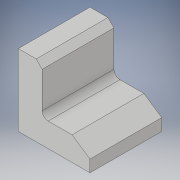
# Autodesk Inventor part: Chamfer
Saved by Autodesk Inventor 2017 (Build 210142000, 142)
## iProperties
Created: 2020-02-03
Part Number: Chamfer
Material: Generic
Document SubType Name: Modeling
Designer: 10042265
Density: 1 g/cm^3
Appearance: Default
Author: 10042265
Autodesk Inventor part; units mm, degrees
ref_plane "YZ Plane" through (0, 0, 0) normal (1, 0, 0) x (0, 1, 0)
ref_plane "XZ Plane" through (0, 0, 0) normal (0, 1, 0) x (-1, 0, 0)
ref_plane "XY Plane" through (0, 0, 0) normal (0, 0, 1) x (1, 0, 0)
sketch "Sketch1" plane through (0, 0, 0) normal (0, 0, 1) x (1, 0, 0)
  line L0 (0, 0) -> (38.1, 0)
  line L1 (38.1, 0) -> (38.1, 12.7)
  line L2 (38.1, 12.7) -> (12.7, 12.7)
  line L3 (12.7, 12.7) -> (12.7, 38.1)
  line L4 (12.7, 38.1) -> (0, 38.1)
  line L5 (0, 38.1) -> (0, 0)
  dimension "d0" = 38.1
  dimension "d1" = 12.7
  dimension "d2" = 25.4
  dimension "d3" = 25.4
  constraints: 12 end point, 4 perpendicular, 1 horizontal, 1 vertical
  measures "d0" distance of L0.start L0.end
  measures "d1" distance of L0.end L1.end
  measures "d2" distance of L1.end L2.end
  measures "d3" distance of L2.end L3.end
extrude "Extrusion1" add sketch "Sketch1" along normal blind 38.1
fillet "Fillet3" radius 3.175 1 edges at (12.7, 12.7, 19.05)
chamfer "Chamfer1" distance 3.175 angle 45 1 edges at (12.7, 38.1, 19.05) measured on face at (8.4667, 38.1, 12.7)
chamfer "Chamfer2" distance 6.35 distance2 9.525 1 edges at (38.1, 12.7, 19.05) measured on face at (38.1, 4.2333, 12.7)
body "Solid1"
